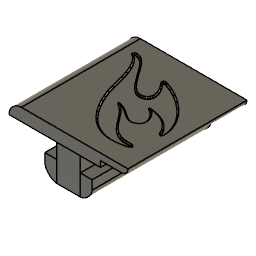
pmmaClip (Autodesk Fusion 360 design; units mm, degrees)
part number: 2026-01-29-15-29-34-594
Autodesk Fusion 360 part; units mm, degrees
note: some values were not read from the file. Chosen so that the rebuilt part matches the saved one: which pieces of a blend or face edit are solid. Set by a fixed rule: which sketch regions a step uses.
sketch "Sketch5" plane through (0, 0, 0) normal (0, 0, 1) x (1, 0, 0)
  line L0 (-20, -20) -> (20, -20)
  line L1 (20, -20) -> (20, 20)
  line L2 (20, 20) -> (-20, 20)
  line L3 (-20, 20) -> (-20, -20)
  line L4 (-20, -20) -> (20, 20) construction
  line L5 (20, -20) -> (-20, 20) construction
  line L6 (-19, 20) -> (-19, -20)
  line L7 (0, 20) -> (0, -20) construction
  line L8 (-10, -20) -> (10, -20) construction
  line L9 (3.95, -20) -> (16.05, -20)
  line L10 (16.05, 20) -> (3.95, 20)
  line L11 (-3.95, 20) -> (-3.95, -20)
  line L12 (3.95, 20) -> (3.95, -20)
  line L13 (10.75, 20) -> (10.75, -20)
  dimension "d29" = 40
  dimension "d30" = 1
  dimension "d100" = 40
  dimension "d101" = 3.95
  dimension "d102" = 9.25
  constraint horizontal L0
  constraint perpendicular L0 L1
  constraint parallel L0 L2
  constraint parallel L1 L3
  constraint coincident L4 origin
  constraint coincident L5 origin
  constraint coincident L2 L6.start
  constraint coincident L0 L6.end
  constraint perpendicular L0 L6
  constraint midpoint L2 L7.start
  constraint midpoint L0 L7.end
  constraint horizontal L8
  constraint coincident L0 L8.start
  constraint horizontal L9
  constraint horizontal L10
  constraint coincident L0 L9.start
  constraint symmetric L7 L9.start L11.end
  constraint symmetric L7 L10.end L11.start
  constraint symmetric L7 L11.start L10.end
  constraint symmetric L7 L11.end L9.start
  constraint coincident L2 L11.start
  constraint coincident L2 L13.start
  constraint coincident L0 L13.end
  constraint perpendicular L0 L13
  measures "d29" distance of L0.end L1.end
  measures "d30" distance of L3 L6
  measures "d100" distance of L1 L3
  measures "d101" distance of L7 L11
  measures "d102" distance of L1 L13
sketch "Sketch6" plane through (0, 0, 0) normal (0, 1, 0) x (1, 0, 0)
  line L0 (0, -56.6756) -> (0, 40) construction
  line L1 (-20, 40) -> (-20, 0) construction
  line L2 (20, 40) -> (20, 0) construction
  line L3 (20, 40) -> (20, 0) construction
  point P0 (0, -4.2)
  point P1 (0, -2.2)
  point P2 (0, -56.6756)
  point P3 (0, 40)
  point P4 (-20, 16)
  point P5 (20, 16)
  point P6 (-20, 12)
  point P7 (-20, 5)
  point P8 (20, 16)
  point P9 (20, 5)
  point P10 (-20, 24)
  point P11 (20, 24)
  point P12 (-31.25, 0)
  point P13 (-19, 0)
  point P14 (20, 24)
  point P15 (20, 12)
  point P16 (19, 0)
  point P17 (20, 16)
  point P18 (31.25, 0)
  point P19 (20, 5)
  dimension "d36" = 40
  dimension "d45" = 20
  dimension "d46" = 20
  dimension "d48" = 40
  dimension "d49" = 12
  dimension "d50" = 5
  dimension "d51" = 16
  dimension "d52" = 8
  dimension "d53" = 16
  dimension "d54" = 12.25
  dimension "d76" = 2
  dimension "d78" = 2.2
  constraint vertical P0 P2
  constraint vertical P1 origin
  constraint coincident P2 L0.start
  constraint coincident P3 L0.end
  constraint vertical L0
  constraint horizontal P4 P17
  constraint horizontal P3 L1.start
  constraint vertical P4 L1.start
  constraint coincident L1 P6
  constraint coincident L1 P7
  constraint symmetric P4 L0 P17
  constraint symmetric L0 L1.start L2.start
  constraint symmetric L0 L1.end L2.end
  constraint symmetric L0 P7 P19
  constraint coincident L1 P10
  constraint symmetric L0 P10 P14
  constraint symmetric L0 P6 P15
  constraint symmetric L0 P12 P18
  constraint symmetric L0 P13 P16
  measures "d36" distance of P3 origin
  measures "d45" distance of P4 L0
  measures "d46" distance of P17 L0
  measures "d48" distance of L1.start L1.end
  measures "d49" distance of L1.end P6
  measures "d50" distance of L1.end P7
  measures "d51" distance of P4 L1.end
  measures "d52" distance of P4 P10
  measures "d53" distance of L1.start P10
  measures "d54" distance of P12 P13
  measures "d76" distance of P0 P1
  measures "d78" distance of P1 origin
extrude "Extrude10" add sketch "Sketch5" along normal up to surface (4.2 mm away) makes body 1
extrude "Extrude14" add sketch "Sketch5" against normal up to surface (12 mm away) contours L0 L2 L11 L12 bodies 1
sketch "Sketch8" plane through (-3.95, 0, 0) normal (1, 0, 0) x (0, 1, 0)
  line L0 (-7.5, -12) -> (7.5, -12)
  line L1 (7.5, -12) -> (7.5, 0)
  line L2 (7.5, 0) -> (-7.5, 0)
  line L3 (-7.5, 0) -> (-7.5, -12)
  line L4 (-7.5, -5) -> (7.5, -5)
  line L5 (7.5, -5) -> (-7.5, -5)
  line L6 (20, -12) -> (-20, -12)
  line L7 (-20, -12) -> (-20, 0)
  line L8 (-20, 0) -> (20, 0)
  line L9 (20, 0) -> (20, -12)
  point P0 (-7.5, 0)
  dimension "d59" = 5
  constraint coincident L3 L4.start
  constraint coincident L1 L4.end
  constraint perpendicular L1 L4
  measures "d59" distance of L4.start P0
extrude "Extrude15" add sketch "Sketch8" along normal blind 4 contours L0 L1 L3 L4 L5 L6 bodies 1
sketch "Sketch9" plane through (-3.95, 0, 0) normal (-1, 0, 0) x (0, -1, 0)
  line L0 (-20, -12) -> (20, -12)
  line L1 (20, -12) -> (20, 0)
  line L2 (20, 0) -> (-20, 0)
  line L3 (-20, 0) -> (-20, -12)
  line L4 (-20, -5) -> (20, -5)
  line L5 (-20, 0) -> (20, 0)
  dimension "d67" = 5
  constraint coincident L3 L4.start
  constraint coincident L1 L4.end
  constraint perpendicular L1 L4
  measures "d67" distance of L4 L5
extrude "Extrude16" add sketch "Sketch9" along normal blind 4 contours L0 L1 L3 L4 bodies 1
fillet "Fillet2" radius 4 tangency weight 0.7 1 edges at (-7.95, 0, -12) on bodies 1
split "Split1" by plane through (0, 0, 0) normal (0, 0, 1) bodies 1 makes body 2 at (-6.6667, 6.6667, 4.2)
mirror "Mirror1" about plane through (0, 0, 0) normal (1, 0, 0) of bodies 1 makes body 3
extrude "Extrude20" cut sketch "Sketch5" along normal blind 2 contours L0 L1 L2 L9 L10 L13 bodies 2
sketch "Sketch10" plane through (0, 0, 4.2) normal (0, 0, 1) x (-1, 0, 0)
  line L0 (20, 20) -> (-20, 20)
  line L1 (-20, -20) -> (20, -20)
  line L2 (11.3931, -13.5759) -> (10.0489, -11.9386)
  line L3 (6.4226, -1.6619) -> (5.7888, 0.4564)
  line L4 (11.8577, -13.9433) -> (11.3931, -13.5759)
  line L5 (-5.8787, -1.7177) -> (-6.6984, -1.6466)
  line L6 (-10.5852, 12.4723) -> (-9.5592, 12.2451)
  line L7 (4.281, 4.0298) -> (3.2238, 5.9796)
  line L8 (8.2073, -12.0995) -> (9.5614, -13.5445)
  line L9 (-6.6984, -1.6466) -> (-9.1386, -1.1205)
  line L10 (1.2334, 1.8927) -> (0.4118, 1.9717)
  line L11 (12.5465, -14.3343) -> (12.4552, -14.1803)
  line L12 (7.5556, -5.9877) -> (6.4226, -1.6619)
  line L13 (-8.8156, 2.108) -> (-8.3751, 1.1952)
  line L14 (-7.5042, 5.2424) -> (-8.4279, 4.6529)
  line L15 (-8.9095, 3.8952) -> (-9.0162, 3.0274)
  line L16 (1.8074, 8.1049) -> (0.001, 10.184)
  line L17 (-2.2261, 11.9949) -> (-3.507, 12.7305)
  line L18 (4.0712, -6.4403) -> (5.4719, -8.3341)
  line L19 (3.2238, 5.9796) -> (1.8074, 8.1049)
  line L20 (10.0489, -11.9386) -> (9.0114, -10.0944)
  line L21 (-4.9045, 13.3159) -> (-6.4227, 13.7234)
  line L22 (0.3802, 2.7933) -> (1.109, 2.2778)
  line L23 (-4.8517, 8.6039) -> (-2.355, 5.3476)
  line L24 (12.2187, -14.0973) -> (11.8577, -13.9433)
  line L25 (-11.7071, 12.5422) -> (-10.5852, 12.4723)
  line L26 (5.4719, -8.3341) -> (8.2073, -12.0995)
  line L27 (-13.6362, 13.112) -> (-13.9034, 12.8898)
  line L28 (-13.7291, 12.6888) -> (-13.2556, 12.5856)
  line L29 (-11.7387, 13.6008) -> (-13.0107, 13.3164)
  line L30 (-1.0575, 3.9096) -> (0.3802, 2.7933)
  line L31 (-1.058, 11.1368) -> (-2.2261, 11.9949)
  line L32 (-2.0299, -3.6276) -> (-1.3016, -3.3638)
  line L33 (-9.8359, 13.8936) -> (-11.7387, 13.6008)
  line L34 (-6.4227, 13.7234) -> (-8.0652, 13.9252)
  line L35 (-9.5592, 12.2451) -> (-7.7543, 11.3922)
  line L36 (9.0114, -10.0944) -> (8.2055, -8.0938)
  line L37 (-3.507, 12.7305) -> (-4.9045, 13.3159)
  line L38 (-8.0652, 13.9252) -> (-9.8359, 13.8936)
  line L39 (12.4552, -14.1803) -> (12.2187, -14.0973)
  line L40 (-13.9034, 12.8898) -> (-13.7291, 12.6888)
  line L41 (8.2055, -8.0938) -> (7.5556, -5.9877)
  line L42 (5.0097, 2.4773) -> (4.281, 4.0298)
  line L43 (-13.0107, 13.3164) -> (-13.6362, 13.112)
  line L44 (-6.212, 10.1297) -> (-4.8517, 8.6039)
  line L45 (0.3961, -3.3842) -> (1.1558, -3.6969)
  line L46 (0.001, 10.184) -> (-1.058, 11.1368)
  line L47 (5.7888, 0.4564) -> (5.0097, 2.4773)
  line L48 (-7.7543, 11.3922) -> (-6.212, 10.1297)
  line L49 (-2.355, 5.3476) -> (-1.0575, 3.9096)
  line L50 (1.109, 2.2778) -> (1.3023, 2.0401)
  line L51 (1.3023, 2.0401) -> (1.2334, 1.8927)
  line L52 (-13.2556, 12.5856) -> (-11.7071, 12.5422)
  line L53 (-5.6378, -1.295) -> (-5.4502, -1.5992)
  line L54 (-9.0162, 3.0274) -> (-8.8156, 2.108)
  line L55 (-10.5399, -5.9305) -> (-8.3362, -7.7081)
  line L56 (-14.1219, -1.6414) -> (-12.5102, -3.8958)
  line L57 (-1.5791, -11.1268) -> (-1.0497, -11.269)
  line L58 (-9.1386, -1.1205) -> (-11.1344, -0.3648)
  line L59 (-3.9076, 4.2648) -> (-4.8315, 4.845)
  line L60 (-6.2876, -0.9198) -> (-5.6378, -1.295)
  line L61 (-7.762, 0.3475) -> (-7.0437, -0.377)
  line L62 (-14.8203, 3.1437) -> (-15.1161, 3.8342)
  line L63 (-15.8014, 4.0692) -> (-15.7678, 3.378)
  line L64 (-8.3362, -7.7081) -> (-6.0246, -9.1915)
  line L65 (-15.7046, 4.4524) -> (-15.8014, 4.0692)
  line L66 (-6.6126, 5.4188) -> (-7.5042, 5.2424)
  line L67 (-15.2495, 0.7956) -> (-14.1219, -1.6414)
  line L68 (-0.7961, 2.3708) -> (-1.9072, 2.9427)
  line L69 (-4.8315, 4.845) -> (-5.7274, 5.258)
  line L70 (-1.1998, -10.3368) -> (-2.2466, -8.9523)
  line L71 (-15.5927, 2.0709) -> (-15.2495, 0.7956)
  line L72 (-15.1161, 3.8342) -> (-15.3822, 4.3322)
  line L73 (-2.2466, -8.9523) -> (-2.9853, -7.4137)
  line L74 (-15.3822, 4.3322) -> (-15.7046, 4.4524)
  line L75 (-0.71, -11.1742) -> (-0.789, -10.797)
  line L76 (-5.7274, 5.258) -> (-6.6126, 5.4188)
  line L77 (-12.5102, -3.8958) -> (-10.5399, -5.9305)
  line L78 (-14.409, 2.4457) -> (-14.8203, 3.1437)
  line L79 (-0.789, -10.797) -> (-1.1998, -10.3368)
  line L80 (0.4118, 1.9717) -> (-0.7961, 2.3708)
  line L81 (-5.4502, -1.5992) -> (-5.8787, -1.7177)
  line L82 (-12.8398, 0.7731) -> (-14.409, 2.4457)
  line L83 (-6.0246, -9.1915) -> (-3.7305, -10.3435)
  line L84 (-7.0437, -0.377) -> (-6.2876, -0.9198)
  line L85 (-2.9853, -7.4137) -> (-2.9853, -7.4137)
  line L86 (-1.9072, 2.9427) -> (-3.9076, 4.2648)
  line L87 (-15.7678, 3.378) -> (-15.5927, 2.0709)
  line L88 (-1.0497, -11.269) -> (-0.71, -11.1742)
  line L89 (-8.3751, 1.1952) -> (-7.762, 0.3475)
  line L90 (-3.7305, -10.3435) -> (-1.5791, -11.1268)
  line L91 (-11.1344, -0.3648) -> (-12.8398, 0.7731)
  line L92 (-8.4279, 4.6529) -> (-8.9095, 3.8952)
  line L93 (12.0824, -14.6641) -> (12.4322, -14.58)
  line L94 (12.4322, -14.58) -> (12.5465, -14.3343)
  line L95 (-2.5752, -4.0395) -> (-2.0299, -3.6276)
  line L96 (1.1558, -3.6969) -> (2.6357, -4.8235)
  line L97 (-0.3782, -3.274) -> (0.3961, -3.3842)
  line L98 (-3.2356, -5.9048) -> (-3.1658, -5.204)
  line L99 (-2.9853, -7.4137) -> (-3.2356, -5.9048)
  line L100 (-1.3016, -3.3638) -> (-0.3782, -3.274)
  line L101 (2.6357, -4.8235) -> (4.0712, -6.4403)
  line L102 (9.5614, -13.5445) -> (10.2392, -14.0643)
  line L103 (10.2392, -14.0643) -> (10.9191, -14.4133)
  line L104 (10.9191, -14.4133) -> (12.0824, -14.6641)
  line L105 (-3.1658, -5.204) -> (-2.9497, -4.5736)
  line L106 (-2.9497, -4.5736) -> (-2.5752, -4.0395)
  line L107 (-20, 20) -> (-20, -20)
  line L108 (20, -20) -> (20, 20)
extrude "Extrude21" cut sketch "Sketch10" against normal blind 0.5 contours L2 L3 L4 L5 L6 L7 L8 L9 L10 L11 L12 L13 L14 L15 L16 L17 L18 L19 L20 L21 L22 L23 L24 L25 L26 L27 L28 L29 L30 L31 L32 L33 L34 L35 L36 L37 L38 L39 L40 L41 L42 L43 L44 L45 L46 L47 L48 L49 L50 L51 L52 L53 L54 L55 L56 L57 L58 L59 L60 L61 L62 L63 L64 L65 L66 L67 L68 L69 L70 L71 L72 L73 L74 L75 L76 L77 L78 L79 L80 L81 L82 L83 L84 L86 L87 L88 L89 L90 L91 L92 L93 L94 L95 L96 L97 L98 L99 L100 L101 L102 L103 L104 L105 L106 bodies 2
chamfer "Chamfer1" distance 0.4 angle 45 104 edges at (1.6657, 3.4957, 4.2) (1.3516, -2.6568, 4.2) (1.3144, 11.1979, 4.2) (1.642, -11.5659, 4.2) (-0.8226, -1.9322, 4.2) (-12.0382, 14.0203, 4.2) (-11.6254, 13.7596, 4.2) (-10.721, 12.7573, 4.2) (-6.1057, 0.6027, 4.2) (1.7062, -4.6286, 4.2) (-5.3993, -1.4669, 4.2) (-0.7446, -2.5356, 4.2) (1.7232, 9.6446, 4.2) (-1.2679, -1.9664, 4.2) (-1.2057, -2.159, 4.2) (2.9074, -3.6037, 4.2) (7.0584, -5.3306, 4.2) (6.17, -5.3384, 4.2) (7.9661, -4.9477, 4.2) (8.6687, -4.2741, 4.2) (13.6244, -1.6094, 4.2) (15.4211, -1.4333, 4.2) (0.1921, -2.1713, 4.2) (8.9628, -3.4613, 4.2) (5.2794, -5.0515, 4.2) (8.9159, -2.5677, 4.2) (3.1105, 6.6593, 4.2) (8.5954, -1.6516, 4.2) (4.3696, -4.5549, 4.2) (9.438, 6.8193, 4.2) (-3.7524, -5.0047, 4.2) (-2.5156, -7.0423, 4.2) (7.4028, 0.0147, 4.2) (-0.9042, -9.1445, 4.2) (5.6636, -13.5196, 4.2) (7.9185, 1.3835, 4.2) (-0.776, 3.5406, 4.2) (5.6645, 1.6584, 4.2) (3.2007, 5.5544, 4.2) (5.9627, 1.1074, 4.2) (14.6146, -2.7947, 4.2) (15.2491, -4.0832, 4.2) (15.7846, -3.7236, 4.2) (-9.5301, 11.0165, 4.2) (5.5319, -9.3668, 4.2) (0.8399, 3.3189, 4.2) (6.6656, 0.6484, 4.2) (-0.009, 3.3291, 4.2) (-3.3535, 5.6319, 4.2) (2.8665, -12.3627, 4.2) (-1.8957, 4.2602, 4.2) (15.5434, -4.3923, 4.2) (0.5285, -10.6604, 4.2) (-4.7715, 7.3872, 4.2) (4.2057, -13.0232, 4.2) (6.9831, -10.761, 4.2) (-7.8805, 7.0408, 4.2) (-8.8843, 12.822, 4.2) (2.3025, 3.8335, 4.2) (7.2439, -13.8243, 4.2) (5.544, 1.4471, 4.2) (6.2886, 1.6821, 4.2) (3.0578, 4.8888, 4.2) (2.7624, 4.3065, 4.2) (14.9682, -3.4889, 4.2) (15.753, -4.2608, 4.2) (-8.6084, 9.0941, 4.2) (0.8799, 11.2216, 4.2) (0.7495, 10.9856, 4.2) (0.9944, 10.5669, 4.2) (8.0685, -0.7714, 4.2) (11.9871, -0.2042, 4.2) (14.6857, 0.4229, 4.2) (10.7873, -13.7472, 4.2) (15.6802, -2.7244, 4.2) (12.3747, -13.4586, 4.2) (10.1365, 0.7426, 4.2) (13.3234, -13.2142, 4.2) (13.7698, -13.0009, 4.2) (-6.8396, 10.2168, 4.2) (13.316, 2.7686, 4.2) (11.525, 4.9131, 4.2) (-9.9003, 13.8044, 4.2) (-12.5008, 14.2573, 4.2) (3.6034, -6.9758, 4.2) (11.1462, -12.5072, 4.2) (-6.9891, 3.8248, 4.2) (13.8162, -12.7893, 4.2) (4.8776, 9.7675, 4.2) (13.4923, -12.6372, 4.2) (12.4813, -12.5639, 4.2) (2.6548, 10.7352, 4.2) (10.0722, -12.3587, 4.2) (-12.4894, 14.4571, 4.2) (0.3386, -3.3514, 4.2) (2.616, 8.183, 4.2) (8.6567, -11.8187, 4.2) (-11.5007, 14.5387, 4.2) (-12.2573, 14.6221, 4.2) (-12.3369, 14.1388, 4.2) (7.1804, 8.4498, 4.2) (-10.5791, 14.2388, 4.2) (-4.6454, -3.2536, 4.2) (8.9505, -13.9094, 4.2) on bodies 2
fillet "Fillet6" radius 4.2 1 edges at (-20, 0, 4.2) on bodies 2
fillet "Fillet7" radius 2.2 1 edges at (20, 0, 2) on bodies 2
equation "d30 = -d83"
equation "d46 = d45"
equation "d47 = 8 mm"
equation "d51 = d48 / 2 - d47 / 2"
equation "d59 = d50"
equation "d67 = d50"
equation "d83 = -1 mm"
equation "d115 = d78 + d76"
equation "d117 = d78"
